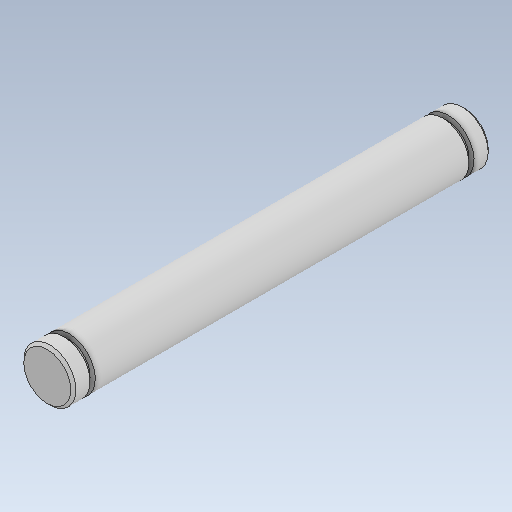
# Autodesk Inventor part: Peça18
Saved by Autodesk Inventor 2021 (Build 250183000, 183)
## iProperties
Category: 41
Created: 2021-07-19
Part Number: Peça18
Material: Genérico
Document SubType Name: Modeling
Designer: Giovanni
Density: 1 g/cm^3
Appearance: Padrão
User Status: 2:1
Author: Giovanni
Keywords: 17
Autodesk Inventor part; units mm, degrees
ref_plane "YZ Plane" through (0, 0, 0) normal (1, 0, 0) x (0, 1, 0)
ref_plane "XZ Plane" through (0, 0, 0) normal (0, 1, 0) x (-1, 0, 0)
ref_plane "XY Plane" through (0, 0, 0) normal (0, 0, 1) x (1, 0, 0)
sketch "Esboço1" plane through (0, 0, 0) normal (0, 0, 1) x (1, 0, 0)
  circle A0 centre (0, 0) radius 5
  dimension "d0" = 10
  constraints: 1 centre point, 1 coincident
  measures "d0" diameter of A0
extrude "Extrusão1" add sketch "Esboço1" along normal mid plane 80
sketch "Esboço2" plane through (0, 0, 0) normal (1, 0, 0) x (0, 1, 0)
  line L0 (5, -40) -> (5, 40) projected
  line L1 (5, 36.8) -> (4, 36.8)
  line L2 (4, 36.8) -> (4, 35.8)
  line L3 (4, 35.8) -> (5, 35.8)
  line L4 (5, 35.8) -> (5, 36.8)
  line L5 (4, -35.8) -> (5, -35.8)
  line L6 (5, -35.8) -> (5, -36.8)
  line L7 (5, -36.8) -> (4, -36.8)
  line L8 (4, -36.8) -> (4, -35.8)
  line L9 (5, 40) -> (-5, 40) projected
  line L10 (-5, -40) -> (5, -40) projected
  line L11 (0, -56) -> (0, 56) projected
  point P0 (0, 0)
  dimension "d3" = 4.2
  dimension "d4" = 1
  dimension "d5" = 4
  dimension "d6" = 1
  dimension "d7" = 4.2
  constraints: 16 end point, 4 parallel, 3 point on line, 2 horizontal, 2 perpendicular
  measures "d3" distance between parallel lines of L3 L9
  measures "d4" distance between parallel lines of L3 L1
  measures "d5" horizontal distance of point (0, 0) L2.end
  measures "d6" distance between parallel lines of L7 L5
  measures "d7" distance between parallel lines of L5 L10
revolve "Revolução1" cut sketch "Esboço2" angle 360 about axis through (0, 0, -10) along (0, 0, 1) contours L7 L8 L5 L0 | L3 L2 L1 L0
chamfer "Chanfro1" distance 0.5 angle 45 2 edges at (-5, 0, 40) (-5, 0, -40)
